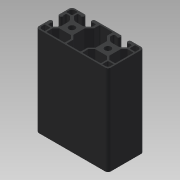
# Autodesk Inventor part: 40-4083-LITE-BLACK-FB
Saved by Autodesk Inventor 2013 (Build 170138000, 138)
## iProperties
Company: 80/20 Inc.
Created: 2014-04-23
Part Number: 40-4083-LITE-BLACK-FB
Material: Generic
Document SubType Name: Modeling
Designer: Ross Bowman
Density: 1 g/cm^3
Engineer: Ross Bowman
Catalog Web Link: 8020.net
Vendor: 80/20 Inc.
Material: 6105-T5 Aluminum
Author: Ross Bowman
Keywords: 80/20 , 8020 , T-Slot , Extrusion
Autodesk Inventor part; units mm, degrees
ref_plane "YZ Plane" through (0, 0, 0) normal (1, 0, 0) x (0, 1, 0)
ref_plane "XZ Plane" through (0, 0, 0) normal (0, 1, 0) x (-1, 0, 0)
ref_plane "XY Plane" through (0, 0, 0) normal (0, 0, 1) x (1, 0, 0)
sketch "Sketch1" plane through (0, 0, 0) normal (0, 0, 1) x (1, 0, 0)
  circle A0 centre (-20, 0) radius 3.3778
  circle A1 centre (20, 0) radius 3.3778
  arc A2 (31.462, -10.0253) -> (32.0906, -10.2857) centre (32.0906, -9.3967) ccw
  line L0 (27.9429, -6.5063) -> (31.462, -10.0253)
  arc A3 (27.6825, -5.8776) -> (27.9429, -6.5063) centre (28.5715, -5.8776) ccw
  line L1 (27.6825, 6.0573) -> (27.6825, -5.8776)
  arc A4 (27.9429, 6.6858) -> (27.6825, 6.0573) centre (28.5714, 6.0573) ccw
  line L2 (31.2824, 10.0254) -> (27.9429, 6.6858)
  arc A5 (31.911, 10.2857) -> (31.2824, 10.0254) centre (31.911, 9.3968) ccw
  line L3 (37.4216, 10.2857) -> (31.911, 10.2857)
  arc A6 (38.3105, 9.3968) -> (37.4216, 10.2857) centre (37.4216, 9.3968) ccw
  line L4 (38.3105, -9.3968) -> (38.3105, 9.3968)
  arc A7 (37.4216, -10.2857) -> (38.3105, -9.3968) centre (37.4216, -9.3968) ccw
  line L5 (32.0906, -10.2857) -> (37.4216, -10.2857)
  arc A8 (26.6858, -7.9429) -> (26.0572, -7.6825) centre (26.0572, -8.5715) ccw
  line L6 (30.0253, -11.2824) -> (26.6858, -7.9429)
  arc A9 (30.2857, -11.911) -> (30.0253, -11.2824) centre (29.3967, -11.911) ccw
  line L7 (30.2857, -17.4603) -> (30.2857, -11.911)
  arc A10 (29.3968, -18.3492) -> (30.2857, -17.4603) centre (29.3968, -17.4603) ccw
  line L8 (10.6032, -18.3492) -> (29.3968, -18.3492)
  arc A11 (9.7143, -17.4603) -> (10.6032, -18.3492) centre (10.6032, -17.4603) ccw
  line L9 (9.7143, -11.911) -> (9.7143, -17.4603)
  arc A12 (9.9746, -11.2824) -> (9.7143, -11.911) centre (10.6032, -11.911) ccw
  line L10 (13.3142, -7.9429) -> (9.9746, -11.2824)
  arc A13 (13.9427, -7.6825) -> (13.3142, -7.9429) centre (13.9427, -8.5714) ccw
  line L11 (26.0572, -7.6825) -> (13.9427, -7.6825)
  arc A14 (-7.8095, -11.122) -> (-8.0699, -10.4935) centre (-8.6984, -11.122) ccw
  line L12 (-12.0571, -6.5062) -> (-8.0699, -10.4935)
  arc A15 (-12.3175, -5.8777) -> (-12.0571, -6.5062) centre (-11.4286, -5.8777) ccw
  line L13 (-12.3175, 6.0573) -> (-12.3175, -5.8777)
  arc A16 (-12.0571, 6.6858) -> (-12.3175, 6.0573) centre (-11.4286, 6.0573) ccw
  line L14 (-7.435, 11.308) -> (-12.0571, 6.6858)
  arc A17 (-7.435, 11.308) -> (-7.1746, 11.9365) centre (-8.0635, 11.9365) ccw
  line L15 (-7.1746, 17.4216) -> (-7.1746, 11.9365)
  arc A18 (-6.2857, 18.3105) -> (-7.1746, 17.4216) centre (-6.2857, 17.4216) ccw
  line L16 (6.2857, 18.3105) -> (-6.2857, 18.3105)
  arc A19 (7.1746, 17.4216) -> (6.2857, 18.3105) centre (6.2857, 17.4216) ccw
  line L17 (7.1746, 11.9365) -> (7.1746, 17.4216)
  arc A20 (7.1746, 11.9365) -> (7.435, 11.308) centre (8.0635, 11.9365) ccw
  line L18 (12.0571, 6.6858) -> (7.435, 11.308)
  arc A21 (12.3175, 6.0573) -> (12.0571, 6.6858) centre (11.4286, 6.0573) ccw
  line L19 (12.3175, -5.8777) -> (12.3175, 6.0573)
  arc A22 (12.0571, -6.5062) -> (12.3175, -5.8777) centre (11.4286, -5.8777) ccw
  line L20 (8.0699, -10.4935) -> (12.0571, -6.5062)
  arc A23 (8.0699, -10.4935) -> (7.8095, -11.122) centre (8.6984, -11.122) ccw
  line L21 (7.8095, -17.4603) -> (7.8095, -11.122)
  arc A24 (6.9206, -18.3492) -> (7.8095, -17.4603) centre (6.9206, -17.4603) ccw
  line L22 (-6.9206, -18.3492) -> (6.9206, -18.3492)
  arc A25 (-7.8095, -17.4603) -> (-6.9206, -18.3492) centre (-6.9206, -17.4603) ccw
  line L23 (-7.8095, -11.122) -> (-7.8095, -17.4603)
  arc A26 (-10.6032, -18.3492) -> (-9.7143, -17.4603) centre (-10.6032, -17.4603) ccw
  line L24 (-29.3968, -18.3492) -> (-10.6032, -18.3492)
  arc A27 (-30.2857, -17.4603) -> (-29.3968, -18.3492) centre (-29.3968, -17.4603) ccw
  line L25 (-30.2857, -11.911) -> (-30.2857, -17.4603)
  arc A28 (-30.0254, -11.2824) -> (-30.2857, -11.911) centre (-29.3968, -11.911) ccw
  line L26 (-26.6858, -7.9429) -> (-30.0254, -11.2824)
  arc A29 (-26.0573, -7.6825) -> (-26.6858, -7.9429) centre (-26.0573, -8.5714) ccw
  line L27 (-13.9427, -7.6825) -> (-26.0573, -7.6825)
  arc A30 (-13.3142, -7.9429) -> (-13.9427, -7.6825) centre (-13.9427, -8.5714) ccw
  line L28 (-9.9746, -11.2824) -> (-13.3142, -7.9429)
  arc A31 (-9.7143, -11.911) -> (-9.9746, -11.2824) centre (-10.6032, -11.911) ccw
  line L29 (-9.7143, -17.4603) -> (-9.7143, -11.911)
  arc A32 (37.9695, 11.9365) -> (38.3495, 12.3165) centre (37.9695, 12.3165) ccw
  line L30 (33.2063, 11.9365) -> (37.9695, 11.9365)
  arc A33 (31.9365, 13.2063) -> (33.2063, 11.9365) centre (33.2063, 13.2063) ccw
  line L31 (31.9365, 17.9693) -> (31.9365, 13.2063)
  arc A34 (32.3165, 18.3492) -> (31.9365, 17.9693) centre (32.3165, 17.9693) ccw
  line L32 (35.5555, 18.3492) -> (32.3165, 18.3492)
  arc A35 (38.3495, 15.5552) -> (35.5555, 18.3492) centre (35.5555, 15.5552) ccw
  line L33 (38.3495, 12.3165) -> (38.3495, 15.5552)
  arc A36 (33.2063, -11.9365) -> (31.9365, -13.2063) centre (33.2063, -13.2063) ccw
  line L34 (37.9695, -11.9365) -> (33.2063, -11.9365)
  arc A37 (38.3495, -12.3165) -> (37.9695, -11.9365) centre (37.9695, -12.3165) ccw
  line L35 (38.3495, -15.5552) -> (38.3495, -12.3165)
  arc A38 (35.5555, -18.3492) -> (38.3495, -15.5552) centre (35.5555, -15.5552) ccw
  line L36 (32.3165, -18.3492) -> (35.5555, -18.3492)
  arc A39 (31.9365, -17.9693) -> (32.3165, -18.3492) centre (32.3165, -17.9693) ccw
  line L37 (31.9365, -13.2063) -> (31.9365, -17.9693)
  arc A40 (-33.2063, 11.9365) -> (-31.9365, 13.2063) centre (-33.2063, 13.2063) ccw
  line L38 (-37.9695, 11.9365) -> (-33.2063, 11.9365)
  arc A41 (-38.3495, 12.3165) -> (-37.9695, 11.9365) centre (-37.9695, 12.3165) ccw
  line L39 (-38.3495, 15.5552) -> (-38.3495, 12.3165)
  arc A42 (-35.5555, 18.3492) -> (-38.3495, 15.5552) centre (-35.5555, 15.5552) ccw
  line L40 (-32.3165, 18.3492) -> (-35.5555, 18.3492)
  arc A43 (-31.9365, 17.9693) -> (-32.3165, 18.3492) centre (-32.3165, 17.9693) ccw
  line L41 (-31.9365, 13.2063) -> (-31.9365, 17.9693)
  arc A44 (-37.9695, -11.9365) -> (-38.3495, -12.3165) centre (-37.9695, -12.3165) ccw
  line L42 (-33.2063, -11.9365) -> (-37.9695, -11.9365)
  arc A45 (-31.9365, -13.2063) -> (-33.2063, -11.9365) centre (-33.2063, -13.2063) ccw
  line L43 (-31.9365, -17.9693) -> (-31.9365, -13.2063)
  arc A46 (-32.3165, -18.3492) -> (-31.9365, -17.9693) centre (-32.3165, -17.9693) ccw
  line L44 (-35.5555, -18.3492) -> (-32.3165, -18.3492)
  arc A47 (-38.3495, -15.5552) -> (-35.5555, -18.3492) centre (-35.5555, -15.5552) ccw
  line L45 (-38.3495, -12.3165) -> (-38.3495, -15.5552)
  arc A48 (40, 16.8254) -> (36.8254, 20) centre (36.8254, 16.8254) ccw
  line L46 (36.8254, 20) -> (25.6381, 20)
  arc A49 (25.6381, 20) -> (24.0635, 18.4254) centre (25.6381, 18.4254) ccw
  line L47 (24.0635, 18.4254) -> (24.0635, 17.5111)
  arc A50 (24.0635, 17.5111) -> (25.6381, 15.9365) centre (25.6381, 17.5111) ccw
  line L48 (25.6381, 15.9365) -> (26.3446, 15.9365)
  arc A51 (26.3446, 15.9365) -> (26.7243, 16.3032) centre (26.3446, 16.3165) ccw
  line L49 (26.7243, 16.3032) -> (26.7253, 16.3317)
  arc A52 (27.105, 16.6984) -> (26.7253, 16.3317) centre (27.105, 16.3185) ccw
  line L50 (27.105, 16.6984) -> (29.0159, 16.6984)
  arc A53 (30.2857, 15.4286) -> (29.0159, 16.6984) centre (29.0159, 15.4286) ccw
  line L51 (30.2857, 15.4286) -> (30.2857, 12.9885)
  arc A54 (30.0254, 12.3599) -> (30.2857, 12.9885) centre (29.3968, 12.9885) ccw
  line L52 (30.0254, 12.3599) -> (26.739, 9.0736)
  arc A55 (23.3808, 7.6825) -> (26.739, 9.0736) centre (23.3808, 12.4317) ccw
  line L53 (23.3808, 7.6825) -> (16.6192, 7.6825)
  arc A56 (13.261, 9.0736) -> (16.6192, 7.6825) centre (16.6192, 12.4317) ccw
  line L54 (13.261, 9.0736) -> (9.9746, 12.3599)
  arc A57 (9.7143, 12.9885) -> (9.9746, 12.3599) centre (10.6032, 12.9885) ccw
  line L55 (9.7143, 12.9885) -> (9.7143, 15.4286)
  arc A58 (10.9841, 16.6984) -> (9.7143, 15.4286) centre (10.9841, 15.4286) ccw
  line L56 (10.9841, 16.6984) -> (12.895, 16.6984)
  arc A59 (13.2747, 16.3317) -> (12.895, 16.6984) centre (12.895, 16.3185) ccw
  line L57 (13.2747, 16.3317) -> (13.2757, 16.3032)
  arc A60 (13.2757, 16.3032) -> (13.6554, 15.9365) centre (13.6554, 16.3165) ccw
  line L58 (13.6554, 15.9365) -> (14.3619, 15.9365)
  arc A61 (14.3619, 15.9365) -> (15.9365, 17.5111) centre (14.3619, 17.5111) ccw
  line L59 (15.9365, 17.5111) -> (15.9365, 18.4254)
  arc A62 (15.9365, 18.4254) -> (14.3619, 20) centre (14.3619, 18.4254) ccw
  line L60 (14.3619, 20) -> (-14.3619, 20)
  arc A63 (-14.3619, 20) -> (-15.9365, 18.4254) centre (-14.3619, 18.4254) ccw
  line L61 (-15.9365, 18.4254) -> (-15.9365, 17.5111)
  arc A64 (-15.9365, 17.5111) -> (-14.3619, 15.9365) centre (-14.3619, 17.5111) ccw
  line L62 (-14.3619, 15.9365) -> (-13.6554, 15.9365)
  arc A65 (-13.6554, 15.9365) -> (-13.2757, 16.3032) centre (-13.6554, 16.3165) ccw
  line L63 (-13.2757, 16.3032) -> (-13.2747, 16.3317)
  arc A66 (-12.895, 16.6984) -> (-13.2747, 16.3317) centre (-12.895, 16.3185) ccw
  line L64 (-12.895, 16.6984) -> (-10.9841, 16.6984)
  arc A67 (-9.7143, 15.4286) -> (-10.9841, 16.6984) centre (-10.9841, 15.4286) ccw
  line L65 (-9.7143, 15.4286) -> (-9.7143, 12.9885)
  arc A68 (-9.9746, 12.3599) -> (-9.7143, 12.9885) centre (-10.6032, 12.9885) ccw
  line L66 (-9.9746, 12.3599) -> (-13.261, 9.0736)
  arc A69 (-16.6192, 7.6825) -> (-13.261, 9.0736) centre (-16.6192, 12.4317) ccw
  line L67 (-16.6192, 7.6825) -> (-23.3808, 7.6825)
  arc A70 (-26.739, 9.0736) -> (-23.3808, 7.6825) centre (-23.3808, 12.4317) ccw
  line L68 (-26.739, 9.0736) -> (-30.0254, 12.3599)
  arc A71 (-30.2857, 12.9885) -> (-30.0254, 12.3599) centre (-29.3968, 12.9885) ccw
  line L69 (-30.2857, 12.9885) -> (-30.2857, 15.4286)
  arc A72 (-29.0159, 16.6984) -> (-30.2857, 15.4286) centre (-29.0159, 15.4286) ccw
  line L70 (-29.0159, 16.6984) -> (-27.105, 16.6984)
  arc A73 (-26.7253, 16.3317) -> (-27.105, 16.6984) centre (-27.105, 16.3185) ccw
  line L71 (-26.7253, 16.3317) -> (-26.7243, 16.3032)
  arc A74 (-26.7243, 16.3032) -> (-26.3446, 15.9365) centre (-26.3446, 16.3165) ccw
  line L72 (-26.3446, 15.9365) -> (-25.6381, 15.9365)
  arc A75 (-25.6381, 15.9365) -> (-24.0635, 17.5111) centre (-25.6381, 17.5111) ccw
  line L73 (-24.0635, 17.5111) -> (-24.0635, 18.4254)
  arc A76 (-24.0635, 18.4254) -> (-25.6381, 20) centre (-25.6381, 18.4254) ccw
  line L74 (-25.6381, 20) -> (-36.8254, 20)
  arc A77 (-36.8254, 20) -> (-40, 16.8254) centre (-36.8254, 16.8254) ccw
  line L75 (-40, 16.8254) -> (-40, 5.6381)
  arc A78 (-40, 5.6381) -> (-38.4254, 4.0635) centre (-38.4254, 5.6381) ccw
  line L76 (-38.4254, 4.0635) -> (-37.5111, 4.0635)
  arc A79 (-37.5111, 4.0635) -> (-35.9365, 5.6381) centre (-37.5111, 5.6381) ccw
  line L77 (-35.9365, 5.6381) -> (-35.9365, 6.3446)
  arc A80 (-35.9365, 6.3446) -> (-36.3032, 6.7243) centre (-36.3165, 6.3446) ccw
  line L78 (-36.3032, 6.7243) -> (-36.3317, 6.7253)
  arc A81 (-36.6984, 7.105) -> (-36.3317, 6.7253) centre (-36.3185, 7.105) ccw
  line L79 (-36.6984, 7.105) -> (-36.6984, 9.0159)
  arc A82 (-35.4286, 10.2857) -> (-36.6984, 9.0159) centre (-35.4286, 9.0159) ccw
  line L80 (-35.4286, 10.2857) -> (-32.9885, 10.2857)
  arc A83 (-32.3599, 10.0254) -> (-32.9885, 10.2857) centre (-32.9885, 9.3968) ccw
  line L81 (-32.3599, 10.0254) -> (-29.0736, 6.739)
  arc A84 (-27.6825, 3.3808) -> (-29.0736, 6.739) centre (-32.4317, 3.3808) ccw
  line L82 (-27.6825, 3.3808) -> (-27.6825, -3.3808)
  arc A85 (-29.0736, -6.739) -> (-27.6825, -3.3808) centre (-32.4317, -3.3808) ccw
  line L83 (-29.0736, -6.739) -> (-32.3599, -10.0254)
  arc A86 (-32.9885, -10.2857) -> (-32.3599, -10.0254) centre (-32.9885, -9.3968) ccw
  line L84 (-32.9885, -10.2857) -> (-35.4286, -10.2857)
  arc A87 (-36.6984, -9.0159) -> (-35.4286, -10.2857) centre (-35.4286, -9.0159) ccw
  line L85 (-36.6984, -9.0159) -> (-36.6984, -7.105)
  arc A88 (-36.3317, -6.7253) -> (-36.6984, -7.105) centre (-36.3185, -7.105) ccw
  line L86 (-36.3317, -6.7253) -> (-36.3032, -6.7243)
  arc A89 (-36.3032, -6.7243) -> (-35.9365, -6.3446) centre (-36.3165, -6.3446) ccw
  line L87 (-35.9365, -6.3446) -> (-35.9365, -5.6381)
  arc A90 (-35.9365, -5.6381) -> (-37.5111, -4.0635) centre (-37.5111, -5.6381) ccw
  line L88 (-37.5111, -4.0635) -> (-38.4254, -4.0635)
  arc A91 (-38.4254, -4.0635) -> (-40, -5.6381) centre (-38.4254, -5.6381) ccw
  line L89 (-40, -5.6381) -> (-40, -16.8254)
  arc A92 (-40, -16.8254) -> (-36.8254, -20) centre (-36.8254, -16.8254) ccw
  line L90 (-36.8254, -20) -> (36.8254, -20)
  arc A93 (36.8254, -20) -> (40, -16.8254) centre (36.8254, -16.8254) ccw
  line L91 (40, -16.8254) -> (40, 16.8254)
  point P0 (0, 0)
  constraints: 184 end point, 184 point on circle, 94 centre point
extrude "Extrusion1" add sketch "Sketch1" against normal blind 100
body "Solid1"
